Autodesk Inventor part; units mm, degrees
(part 2 of 2)
sketch "Sketch8" plane through (0, 0, -1) normal (0, 0, -1) x (-1, 0, 0)
  line L0 (0.5, -44.4972) -> (0.5, -45.4972)
  line L1 (0.5, -45.4972) -> (-0.5, -45.4972)
  line L2 (-0.5, -45.4972) -> (-0.5, -44.4972)
  arc A0 (-1.3127, -44.4806) -> (1.3127, -44.4806) centre (0, 0) ccw construction
  arc A1 (-0.5, -44.4972) -> (0.5, -44.4972) centre (0, 0) ccw
  line L3 (4.1728, -44.3039) -> (4.2554, -45.3005)
  line L4 (4.2554, -45.3005) -> (3.2588, -45.3831)
  line L5 (3.2588, -45.3831) -> (3.1763, -44.3865)
  arc A2 (3.1763, -44.3865) -> (4.1728, -44.3039) centre (0, 0) ccw
  line L6 (7.8172, -43.808) -> (7.9818, -44.7944)
  line L7 (7.9818, -44.7944) -> (6.9954, -44.959)
  line L8 (6.9954, -44.959) -> (6.8308, -43.9726)
  arc A3 (6.8308, -43.9726) -> (7.8172, -43.808) centre (0, 0) ccw
  line L9 (11.4081, -43.0128) -> (11.6536, -43.9822)
  line L10 (11.6536, -43.9822) -> (10.6842, -44.2277)
  line L11 (10.6842, -44.2277) -> (10.4387, -43.2583)
  arc A4 (10.4387, -43.2583) -> (11.4081, -43.0128) centre (0, 0) ccw
  line L12 (14.9211, -41.9239) -> (15.2458, -42.8697)
  line L13 (15.2458, -42.8697) -> (14.3, -43.1944)
  line L14 (14.3, -43.1944) -> (13.9753, -42.2486)
  arc A5 (13.9753, -42.2486) -> (14.9211, -41.9239) centre (0, 0) ccw
  line L15 (18.3322, -40.5485) -> (18.7339, -41.4643)
  line L16 (18.7339, -41.4643) -> (17.8181, -41.866)
  line L17 (17.8181, -41.866) -> (17.4164, -40.9502)
  arc A6 (17.4164, -40.9502) -> (18.3322, -40.5485) centre (0, 0) ccw
  line L18 (21.6181, -38.8961) -> (22.094, -39.7756)
  line L19 (22.094, -39.7756) -> (21.2145, -40.2516)
  line L20 (21.2145, -40.2516) -> (20.7386, -39.3721)
  arc A7 (20.7386, -39.3721) -> (21.6181, -38.8961) centre (0, 0) ccw
  line L21 (24.7562, -36.9781) -> (25.3032, -37.8152)
  line L22 (25.3032, -37.8152) -> (24.466, -38.3622)
  line L23 (24.466, -38.3622) -> (23.9191, -37.525)
  arc A8 (23.9191, -37.525) -> (24.7562, -36.9781) centre (0, 0) ccw
  line L24 (27.7253, -34.8074) -> (28.3395, -35.5966)
  line L25 (28.3395, -35.5966) -> (27.5504, -36.2108)
  line L26 (27.5504, -36.2108) -> (26.9362, -35.4216)
  arc A9 (26.9362, -35.4216) -> (27.7253, -34.8074) centre (0, 0) ccw
  line L27 (30.505, -32.399) -> (31.1823, -33.1347)
  line L28 (31.1823, -33.1347) -> (30.4465, -33.812)
  line L29 (30.4465, -33.812) -> (29.7693, -33.0763)
  arc A10 (29.7693, -33.0763) -> (30.505, -32.399) centre (0, 0) ccw
  line L30 (33.0763, -29.7693) -> (33.812, -30.4465)
  line L31 (33.812, -30.4465) -> (33.1347, -31.1823)
  line L32 (33.1347, -31.1823) -> (32.399, -30.505)
  arc A11 (32.399, -30.505) -> (33.0763, -29.7693) centre (0, 0) ccw
  line L33 (35.4216, -26.9362) -> (36.2108, -27.5504)
  line L34 (36.2108, -27.5504) -> (35.5966, -28.3395)
  line L35 (35.5966, -28.3395) -> (34.8074, -27.7253)
  arc A12 (34.8074, -27.7253) -> (35.4216, -26.9362) centre (0, 0) ccw
  line L36 (37.525, -23.9191) -> (38.3622, -24.466)
  line L37 (38.3622, -24.466) -> (37.8152, -25.3032)
  line L38 (37.8152, -25.3032) -> (36.9781, -24.7562)
  arc A13 (36.9781, -24.7562) -> (37.525, -23.9191) centre (0, 0) ccw
  line L39 (39.3721, -20.7386) -> (40.2516, -21.2145)
  line L40 (40.2516, -21.2145) -> (39.7756, -22.094)
  line L41 (39.7756, -22.094) -> (38.8961, -21.6181)
  arc A14 (38.8961, -21.6181) -> (39.3721, -20.7386) centre (0, 0) ccw
  line L42 (40.9502, -17.4164) -> (41.866, -17.8181)
  line L43 (41.866, -17.8181) -> (41.4643, -18.7339)
  line L44 (41.4643, -18.7339) -> (40.5485, -18.3322)
  arc A15 (40.5485, -18.3322) -> (40.9502, -17.4164) centre (0, 0) ccw
  line L45 (42.2486, -13.9753) -> (43.1944, -14.3)
  line L46 (43.1944, -14.3) -> (42.8697, -15.2458)
  line L47 (42.8697, -15.2458) -> (41.9239, -14.9211)
  arc A16 (41.9239, -14.9211) -> (42.2486, -13.9753) centre (0, 0) ccw
  line L48 (43.2583, -10.4387) -> (44.2277, -10.6842)
  line L49 (44.2277, -10.6842) -> (43.9822, -11.6536)
  line L50 (43.9822, -11.6536) -> (43.0128, -11.4081)
  arc A17 (43.0128, -11.4081) -> (43.2583, -10.4387) centre (0, 0) ccw
  line L51 (43.9726, -6.8308) -> (44.959, -6.9954)
  line L52 (44.959, -6.9954) -> (44.7944, -7.9818)
  line L53 (44.7944, -7.9818) -> (43.808, -7.8172)
  arc A18 (43.808, -7.8172) -> (43.9726, -6.8308) centre (0, 0) ccw
  line L54 (44.3865, -3.1763) -> (45.3831, -3.2588)
  line L55 (45.3831, -3.2588) -> (45.3005, -4.2554)
  line L56 (45.3005, -4.2554) -> (44.3039, -4.1728)
  arc A19 (44.3039, -4.1728) -> (44.3865, -3.1763) centre (0, 0) ccw
  line L57 (44.4972, 0.5) -> (45.4972, 0.5)
  line L58 (45.4972, 0.5) -> (45.4972, -0.5)
  line L59 (45.4972, -0.5) -> (44.4972, -0.5)
  arc A20 (44.4972, -0.5) -> (44.4972, 0.5) centre (0, 0) ccw
  line L60 (44.3039, 4.1728) -> (45.3005, 4.2554)
  line L61 (45.3005, 4.2554) -> (45.3831, 3.2588)
  line L62 (45.3831, 3.2588) -> (44.3865, 3.1763)
  arc A21 (44.3865, 3.1763) -> (44.3039, 4.1728) centre (0, 0) ccw
  line L63 (43.808, 7.8172) -> (44.7944, 7.9818)
  line L64 (44.7944, 7.9818) -> (44.959, 6.9954)
  line L65 (44.959, 6.9954) -> (43.9726, 6.8308)
  arc A22 (43.9726, 6.8308) -> (43.808, 7.8172) centre (0, 0) ccw
  line L66 (43.0128, 11.4081) -> (43.9822, 11.6536)
  line L67 (43.9822, 11.6536) -> (44.2277, 10.6842)
  line L68 (44.2277, 10.6842) -> (43.2583, 10.4387)
  arc A23 (43.2583, 10.4387) -> (43.0128, 11.4081) centre (0, 0) ccw
  line L69 (41.9239, 14.9211) -> (42.8697, 15.2458)
  line L70 (42.8697, 15.2458) -> (43.1944, 14.3)
  line L71 (43.1944, 14.3) -> (42.2486, 13.9753)
  arc A24 (42.2486, 13.9753) -> (41.9239, 14.9211) centre (0, 0) ccw
  line L72 (40.5485, 18.3322) -> (41.4643, 18.7339)
  line L73 (41.4643, 18.7339) -> (41.866, 17.8181)
  line L74 (41.866, 17.8181) -> (40.9502, 17.4164)
  arc A25 (40.9502, 17.4164) -> (40.5485, 18.3322) centre (0, 0) ccw
  line L75 (38.8961, 21.6181) -> (39.7756, 22.094)
  line L76 (39.7756, 22.094) -> (40.2516, 21.2145)
  line L77 (40.2516, 21.2145) -> (39.3721, 20.7386)
  arc A26 (39.3721, 20.7386) -> (38.8961, 21.6181) centre (0, 0) ccw
  line L78 (36.9781, 24.7562) -> (37.8152, 25.3032)
  line L79 (37.8152, 25.3032) -> (38.3622, 24.466)
  line L80 (38.3622, 24.466) -> (37.525, 23.9191)
  arc A27 (37.525, 23.9191) -> (36.9781, 24.7562) centre (0, 0) ccw
  line L81 (34.8074, 27.7253) -> (35.5966, 28.3395)
  line L82 (35.5966, 28.3395) -> (36.2108, 27.5504)
  line L83 (36.2108, 27.5504) -> (35.4216, 26.9362)
  arc A28 (35.4216, 26.9362) -> (34.8074, 27.7253) centre (0, 0) ccw
  line L84 (32.399, 30.505) -> (33.1347, 31.1823)
  line L85 (33.1347, 31.1823) -> (33.812, 30.4465)
  line L86 (33.812, 30.4465) -> (33.0763, 29.7693)
  arc A29 (33.0763, 29.7693) -> (32.399, 30.505) centre (0, 0) ccw
  line L87 (29.7693, 33.0763) -> (30.4465, 33.812)
  line L88 (30.4465, 33.812) -> (31.1823, 33.1347)
  line L89 (31.1823, 33.1347) -> (30.505, 32.399)
  arc A30 (30.505, 32.399) -> (29.7693, 33.0763) centre (0, 0) ccw
  line L90 (26.9362, 35.4216) -> (27.5504, 36.2108)
  line L91 (27.5504, 36.2108) -> (28.3395, 35.5966)
  line L92 (28.3395, 35.5966) -> (27.7253, 34.8074)
  arc A31 (27.7253, 34.8074) -> (26.9362, 35.4216) centre (0, 0) ccw
  line L93 (23.9191, 37.525) -> (24.466, 38.3622)
  line L94 (24.466, 38.3622) -> (25.3032, 37.8152)
  line L95 (25.3032, 37.8152) -> (24.7562, 36.9781)
  arc A32 (24.7562, 36.9781) -> (23.9191, 37.525) centre (0, 0) ccw
  line L96 (20.7386, 39.3721) -> (21.2145, 40.2516)
  line L97 (21.2145, 40.2516) -> (22.094, 39.7756)
  line L98 (22.094, 39.7756) -> (21.6181, 38.8961)
  arc A33 (21.6181, 38.8961) -> (20.7386, 39.3721) centre (0, 0) ccw
  line L99 (17.4164, 40.9502) -> (17.8181, 41.866)
  line L100 (17.8181, 41.866) -> (18.7339, 41.4643)
  line L101 (18.7339, 41.4643) -> (18.3322, 40.5485)
  arc A34 (18.3322, 40.5485) -> (17.4164, 40.9502) centre (0, 0) ccw
  line L102 (13.9753, 42.2486) -> (14.3, 43.1944)
  line L103 (14.3, 43.1944) -> (15.2458, 42.8697)
  line L104 (15.2458, 42.8697) -> (14.9211, 41.9239)
  arc A35 (14.9211, 41.9239) -> (13.9753, 42.2486) centre (0, 0) ccw
  line L105 (10.4387, 43.2583) -> (10.6842, 44.2277)
  line L106 (10.6842, 44.2277) -> (11.6536, 43.9822)
  line L107 (11.6536, 43.9822) -> (11.4081, 43.0128)
  arc A36 (11.4081, 43.0128) -> (10.4387, 43.2583) centre (0, 0) ccw
  line L108 (6.8308, 43.9726) -> (6.9954, 44.959)
  line L109 (6.9954, 44.959) -> (7.9818, 44.7944)
  line L110 (7.9818, 44.7944) -> (7.8172, 43.808)
  arc A37 (7.8172, 43.808) -> (6.8308, 43.9726) centre (0, 0) ccw
  line L111 (3.1763, 44.3865) -> (3.2588, 45.3831)
  line L112 (3.2588, 45.3831) -> (4.2554, 45.3005)
  line L113 (4.2554, 45.3005) -> (4.1728, 44.3039)
  arc A38 (4.1728, 44.3039) -> (3.1763, 44.3865) centre (0, 0) ccw
  line L114 (-0.5, 44.4972) -> (-0.5, 45.4972)
  line L115 (-0.5, 45.4972) -> (0.5, 45.4972)
  line L116 (0.5, 45.4972) -> (0.5, 44.4972)
  arc A39 (0.5, 44.4972) -> (-0.5, 44.4972) centre (0, 0) ccw
  line L117 (-4.1728, 44.3039) -> (-4.2554, 45.3005)
  line L118 (-4.2554, 45.3005) -> (-3.2588, 45.3831)
  line L119 (-3.2588, 45.3831) -> (-3.1763, 44.3865)
  arc A40 (-3.1763, 44.3865) -> (-4.1728, 44.3039) centre (0, 0) ccw
  line L120 (-7.8172, 43.808) -> (-7.9818, 44.7944)
  line L121 (-7.9818, 44.7944) -> (-6.9954, 44.959)
  line L122 (-6.9954, 44.959) -> (-6.8308, 43.9726)
  arc A41 (-6.8308, 43.9726) -> (-7.8172, 43.808) centre (0, 0) ccw
  line L123 (-11.4081, 43.0128) -> (-11.6536, 43.9822)
  line L124 (-11.6536, 43.9822) -> (-10.6842, 44.2277)
  line L125 (-10.6842, 44.2277) -> (-10.4387, 43.2583)
  arc A42 (-10.4387, 43.2583) -> (-11.4081, 43.0128) centre (0, 0) ccw
  line L126 (-14.9211, 41.9239) -> (-15.2458, 42.8697)
  line L127 (-15.2458, 42.8697) -> (-14.3, 43.1944)
  line L128 (-14.3, 43.1944) -> (-13.9753, 42.2486)
  arc A43 (-13.9753, 42.2486) -> (-14.9211, 41.9239) centre (0, 0) ccw
  line L129 (-18.3322, 40.5485) -> (-18.7339, 41.4643)
  line L130 (-18.7339, 41.4643) -> (-17.8181, 41.866)
  line L131 (-17.8181, 41.866) -> (-17.4164, 40.9502)
  arc A44 (-17.4164, 40.9502) -> (-18.3322, 40.5485) centre (0, 0) ccw
  line L132 (-21.6181, 38.8961) -> (-22.094, 39.7756)
  line L133 (-22.094, 39.7756) -> (-21.2145, 40.2516)
  line L134 (-21.2145, 40.2516) -> (-20.7386, 39.3721)
  arc A45 (-20.7386, 39.3721) -> (-21.6181, 38.8961) centre (0, 0) ccw
  line L135 (-24.7562, 36.9781) -> (-25.3032, 37.8152)
  line L136 (-25.3032, 37.8152) -> (-24.466, 38.3622)
  line L137 (-24.466, 38.3622) -> (-23.9191, 37.525)
  arc A46 (-23.9191, 37.525) -> (-24.7562, 36.9781) centre (0, 0) ccw
  line L138 (-27.7253, 34.8074) -> (-28.3395, 35.5966)
  line L139 (-28.3395, 35.5966) -> (-27.5504, 36.2108)
  line L140 (-27.5504, 36.2108) -> (-26.9362, 35.4216)
  arc A47 (-26.9362, 35.4216) -> (-27.7253, 34.8074) centre (0, 0) ccw
  line L141 (-30.505, 32.399) -> (-31.1823, 33.1347)
  line L142 (-31.1823, 33.1347) -> (-30.4465, 33.812)
  line L143 (-30.4465, 33.812) -> (-29.7693, 33.0763)
  arc A48 (-29.7693, 33.0763) -> (-30.505, 32.399) centre (0, 0) ccw
  line L144 (-33.0763, 29.7693) -> (-33.812, 30.4465)
  line L145 (-33.812, 30.4465) -> (-33.1347, 31.1823)
  line L146 (-33.1347, 31.1823) -> (-32.399, 30.505)
  arc A49 (-32.399, 30.505) -> (-33.0763, 29.7693) centre (0, 0) ccw
  line L147 (-35.4216, 26.9362) -> (-36.2108, 27.5504)
  line L148 (-36.2108, 27.5504) -> (-35.5966, 28.3395)
  line L149 (-35.5966, 28.3395) -> (-34.8074, 27.7253)
  arc A50 (-34.8074, 27.7253) -> (-35.4216, 26.9362) centre (0, 0) ccw
  line L150 (-37.525, 23.9191) -> (-38.3622, 24.466)
  line L151 (-38.3622, 24.466) -> (-37.8152, 25.3032)
  line L152 (-37.8152, 25.3032) -> (-36.9781, 24.7562)
  arc A51 (-36.9781, 24.7562) -> (-37.525, 23.9191) centre (0, 0) ccw
  line L153 (-39.3721, 20.7386) -> (-40.2516, 21.2145)
  line L154 (-40.2516, 21.2145) -> (-39.7756, 22.094)
  line L155 (-39.7756, 22.094) -> (-38.8961, 21.6181)
  arc A52 (-38.8961, 21.6181) -> (-39.3721, 20.7386) centre (0, 0) ccw
  line L156 (-40.9502, 17.4164) -> (-41.866, 17.8181)
  line L157 (-41.866, 17.8181) -> (-41.4643, 18.7339)
  line L158 (-41.4643, 18.7339) -> (-40.5485, 18.3322)
  arc A53 (-40.5485, 18.3322) -> (-40.9502, 17.4164) centre (0, 0) ccw
  line L159 (-42.2486, 13.9753) -> (-43.1944, 14.3)
  line L160 (-43.1944, 14.3) -> (-42.8697, 15.2458)
  line L161 (-42.8697, 15.2458) -> (-41.9239, 14.9211)
  arc A54 (-41.9239, 14.9211) -> (-42.2486, 13.9753) centre (0, 0) ccw
  line L162 (-43.2583, 10.4387) -> (-44.2277, 10.6842)
  line L163 (-44.2277, 10.6842) -> (-43.9822, 11.6536)
  line L164 (-43.9822, 11.6536) -> (-43.0128, 11.4081)
  arc A55 (-43.0128, 11.4081) -> (-43.2583, 10.4387) centre (0, 0) ccw
  line L165 (-43.9726, 6.8308) -> (-44.959, 6.9954)
  line L166 (-44.959, 6.9954) -> (-44.7944, 7.9818)
  line L167 (-44.7944, 7.9818) -> (-43.808, 7.8172)
  arc A56 (-43.808, 7.8172) -> (-43.9726, 6.8308) centre (0, 0) ccw
  line L168 (-44.3865, 3.1763) -> (-45.3831, 3.2588)
  line L169 (-45.3831, 3.2588) -> (-45.3005, 4.2554)
  line L170 (-45.3005, 4.2554) -> (-44.3039, 4.1728)
  arc A57 (-44.3039, 4.1728) -> (-44.3865, 3.1763) centre (0, 0) ccw
  line L171 (-44.4972, -0.5) -> (-45.4972, -0.5)
  line L172 (-45.4972, -0.5) -> (-45.4972, 0.5)
  line L173 (-45.4972, 0.5) -> (-44.4972, 0.5)
  arc A58 (-44.4972, 0.5) -> (-44.4972, -0.5) centre (0, 0) ccw
  line L174 (-44.3039, -4.1728) -> (-45.3005, -4.2554)
  line L175 (-45.3005, -4.2554) -> (-45.3831, -3.2588)
  line L176 (-45.3831, -3.2588) -> (-44.3865, -3.1763)
  arc A59 (-44.3865, -3.1763) -> (-44.3039, -4.1728) centre (0, 0) ccw
  line L177 (-43.808, -7.8172) -> (-44.7944, -7.9818)
  line L178 (-44.7944, -7.9818) -> (-44.959, -6.9954)
  line L179 (-44.959, -6.9954) -> (-43.9726, -6.8308)
  arc A60 (-43.9726, -6.8308) -> (-43.808, -7.8172) centre (0, 0) ccw
  line L180 (-43.0128, -11.4081) -> (-43.9822, -11.6536)
  line L181 (-43.9822, -11.6536) -> (-44.2277, -10.6842)
  line L182 (-44.2277, -10.6842) -> (-43.2583, -10.4387)
  arc A61 (-43.2583, -10.4387) -> (-43.0128, -11.4081) centre (0, 0) ccw
  line L183 (-41.9239, -14.9211) -> (-42.8697, -15.2458)
  line L184 (-42.8697, -15.2458) -> (-43.1944, -14.3)
  line L185 (-43.1944, -14.3) -> (-42.2486, -13.9753)
  arc A62 (-42.2486, -13.9753) -> (-41.9239, -14.9211) centre (0, 0) ccw
  line L186 (-40.5485, -18.3322) -> (-41.4643, -18.7339)
  line L187 (-41.4643, -18.7339) -> (-41.866, -17.8181)
  line L188 (-41.866, -17.8181) -> (-40.9502, -17.4164)
  arc A63 (-40.9502, -17.4164) -> (-40.5485, -18.3322) centre (0, 0) ccw
  line L189 (-38.8961, -21.6181) -> (-39.7756, -22.094)
  line L190 (-39.7756, -22.094) -> (-40.2516, -21.2145)
  line L191 (-40.2516, -21.2145) -> (-39.3721, -20.7386)
  arc A64 (-39.3721, -20.7386) -> (-38.8961, -21.6181) centre (0, 0) ccw
  line L192 (-36.9781, -24.7562) -> (-37.8152, -25.3032)
  line L193 (-37.8152, -25.3032) -> (-38.3622, -24.466)
  line L194 (-38.3622, -24.466) -> (-37.525, -23.9191)
  arc A65 (-37.525, -23.9191) -> (-36.9781, -24.7562) centre (0, 0) ccw
  line L195 (-34.8074, -27.7253) -> (-35.5966, -28.3395)
  line L196 (-35.5966, -28.3395) -> (-36.2108, -27.5504)
  line L197 (-36.2108, -27.5504) -> (-35.4216, -26.9362)
  arc A66 (-35.4216, -26.9362) -> (-34.8074, -27.7253) centre (0, 0) ccw
  line L198 (-32.399, -30.505) -> (-33.1347, -31.1823)
  line L199 (-33.1347, -31.1823) -> (-33.812, -30.4465)
  line L200 (-33.812, -30.4465) -> (-33.0763, -29.7693)
  arc A67 (-33.0763, -29.7693) -> (-32.399, -30.505) centre (0, 0) ccw
  line L201 (-29.7693, -33.0763) -> (-30.4465, -33.812)
  line L202 (-30.4465, -33.812) -> (-31.1823, -33.1347)
  line L203 (-31.1823, -33.1347) -> (-30.505, -32.399)
  arc A68 (-30.505, -32.399) -> (-29.7693, -33.0763) centre (0, 0) ccw
  line L204 (-26.9362, -35.4216) -> (-27.5504, -36.2108)
  line L205 (-27.5504, -36.2108) -> (-28.3395, -35.5966)
  line L206 (-28.3395, -35.5966) -> (-27.7253, -34.8074)
  arc A69 (-27.7253, -34.8074) -> (-26.9362, -35.4216) centre (0, 0) ccw
  line L207 (-23.9191, -37.525) -> (-24.466, -38.3622)
  line L208 (-24.466, -38.3622) -> (-25.3032, -37.8152)
  line L209 (-25.3032, -37.8152) -> (-24.7562, -36.9781)
  arc A70 (-24.7562, -36.9781) -> (-23.9191, -37.525) centre (0, 0) ccw
  line L210 (-20.7386, -39.3721) -> (-21.2145, -40.2516)
  line L211 (-21.2145, -40.2516) -> (-22.094, -39.7756)
  line L212 (-22.094, -39.7756) -> (-21.6181, -38.8961)
  arc A71 (-21.6181, -38.8961) -> (-20.7386, -39.3721) centre (0, 0) ccw
  line L213 (-17.4164, -40.9502) -> (-17.8181, -41.866)
  line L214 (-17.8181, -41.866) -> (-18.7339, -41.4643)
  line L215 (-18.7339, -41.4643) -> (-18.3322, -40.5485)
  arc A72 (-18.3322, -40.5485) -> (-17.4164, -40.9502) centre (0, 0) ccw
  line L216 (-13.9753, -42.2486) -> (-14.3, -43.1944)
  line L217 (-14.3, -43.1944) -> (-15.2458, -42.8697)
  line L218 (-15.2458, -42.8697) -> (-14.9211, -41.9239)
  arc A73 (-14.9211, -41.9239) -> (-13.9753, -42.2486) centre (0, 0) ccw
  line L219 (-10.4387, -43.2583) -> (-10.6842, -44.2277)
  line L220 (-10.6842, -44.2277) -> (-11.6536, -43.9822)
  line L221 (-11.6536, -43.9822) -> (-11.4081, -43.0128)
  arc A74 (-11.4081, -43.0128) -> (-10.4387, -43.2583) centre (0, 0) ccw
  line L222 (-6.8308, -43.9726) -> (-6.9954, -44.959)
  line L223 (-6.9954, -44.959) -> (-7.9818, -44.7944)
  line L224 (-7.9818, -44.7944) -> (-7.8172, -43.808)
  arc A75 (-7.8172, -43.808) -> (-6.8308, -43.9726) centre (0, 0) ccw
  line L225 (-3.1763, -44.3865) -> (-3.2588, -45.3831)
  line L226 (-3.2588, -45.3831) -> (-4.2554, -45.3005)
  line L227 (-4.2554, -45.3005) -> (-4.1728, -44.3039)
  arc A76 (-4.1728, -44.3039) -> (-3.1763, -44.3865) centre (0, 0) ccw
  point P0 (0, 0)
  point P1 (0, -45.4972)
  point P2 (0, -44.5)
  point P3 (3.7571, -45.3418)
  point P4 (7.4886, -44.8767)
  point P5 (11.1689, -44.105)
  point P6 (14.7729, -43.032)
  point P7 (18.276, -41.6651)
  point P8 (21.6543, -40.0136)
  point P9 (24.8846, -38.0887)
  point P10 (27.945, -35.9037)
  point P11 (30.8144, -33.4734)
  point P12 (33.4734, -30.8144)
  point P13 (35.9037, -27.945)
  point P14 (38.0887, -24.8846)
  point P15 (40.0136, -21.6543)
  point P16 (41.6651, -18.276)
  point P17 (43.032, -14.7729)
  point P18 (44.105, -11.1689)
  point P19 (44.8767, -7.4886)
  point P20 (45.3418, -3.7571)
  point P21 (45.4972, 0)
  point P22 (45.3418, 3.7571)
  point P23 (44.8767, 7.4886)
  point P24 (44.105, 11.1689)
  point P25 (43.032, 14.7729)
  point P26 (41.6651, 18.276)
  point P27 (40.0136, 21.6543)
  point P28 (38.0887, 24.8846)
  point P29 (35.9037, 27.945)
  point P30 (33.4734, 30.8144)
  point P31 (30.8144, 33.4734)
  point P32 (27.945, 35.9037)
  point P33 (24.8846, 38.0887)
  point P34 (21.6543, 40.0136)
  point P35 (18.276, 41.6651)
  point P36 (14.7729, 43.032)
  point P37 (11.1689, 44.105)
  point P38 (7.4886, 44.8767)
  point P39 (3.7571, 45.3418)
  point P40 (0, 45.4972)
  point P41 (-3.7571, 45.3418)
  point P42 (-7.4886, 44.8767)
  point P43 (-11.1689, 44.105)
  point P44 (-14.7729, 43.032)
  point P45 (-18.276, 41.6651)
  point P46 (-21.6543, 40.0136)
  point P47 (-24.8846, 38.0887)
  point P48 (-27.945, 35.9037)
  point P49 (-30.8144, 33.4734)
  point P50 (-33.4734, 30.8144)
  point P51 (-35.9037, 27.945)
  point P52 (-38.0887, 24.8846)
  point P53 (-40.0136, 21.6543)
  point P54 (-41.6651, 18.276)
  point P55 (-43.032, 14.7729)
  point P56 (-44.105, 11.1689)
  point P57 (-44.8767, 7.4886)
  point P58 (-45.3418, 3.7571)
  point P59 (-45.4972, 0)
  point P60 (-45.3418, -3.7571)
  point P61 (-44.8767, -7.4886)
  point P62 (-44.105, -11.1689)
  point P63 (-43.032, -14.7729)
  point P64 (-41.6651, -18.276)
  point P65 (-40.0136, -21.6543)
  point P66 (-38.0887, -24.8846)
  point P67 (-35.9037, -27.945)
  point P68 (-33.4734, -30.8144)
  point P69 (-30.8144, -33.4734)
  point P70 (-27.945, -35.9037)
  point P71 (-24.8846, -38.0887)
  point P72 (-21.6543, -40.0136)
  point P73 (-18.276, -41.6651)
  point P74 (-14.7729, -43.032)
  point P75 (-11.1689, -44.105)
  point P76 (-7.4886, -44.8767)
  point P77 (-3.7571, -45.3418)
  dimension "d59" = 1
  dimension "d60" = 1
  dimension "d63" = 360
  constraints: 456 end point, 155 point on circle, 76 centre point, 2 coincident, 2 vertical, 1 concentric, 1 horizontal, 1 midpoint, 1 vertical alignment, 759 other
  measures "d59" distance of L0.start L0.end
  measures "d60" distance of L0.end L1.end
extrude "Extrusion9" add sketch "Sketch8" against normal blind 6
sketch "Sketch9" plane through (0, 0, -1) normal (0, 0, -1) x (-1, 0, 0)
  arc A0 (38.8961, 21.6181) -> (37.525, 23.9191) centre (0, 0) ccw projected
  circle A1 centre (0, 0) radius 44.5
  circle A2 centre (0, 0) radius 49.5
  point P0 (0, 0)
  dimension "d67" = 89
  dimension "d68" = 5
  constraints: 2 centre point, 1 coincident
  measures "d67" diameter of A1
  measures "d68" radial gap between concentric circles of A1 A2
extrude "Extrusion10" cut sketch "Sketch9" against normal blind 2
body "Solid1"
